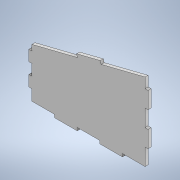
# Autodesk Inventor part: glass_separator
Saved by Autodesk Inventor 2020 (Build 240168000, 168)
## iProperties
Created: 2020-02-26
Part Number: glass_separator
Material: Generic
Document SubType Name: Modeling
Designer: udvarhelyi
Density: 1 g/cm^3
Appearance: Default
Author: udvarhelyi
Autodesk Inventor part; units mm, degrees
ref_plane "YZ Plane" through (0, 0, 0) normal (1, 0, 0) x (0, 1, 0)
ref_plane "XZ Plane" through (0, 0, 0) normal (0, 1, 0) x (-1, 0, 0)
ref_plane "XY Plane" through (0, 0, 0) normal (0, 0, 1) x (1, 0, 0)
sketch "Sketch1" plane through (0, 0, 0) normal (0, 0, 1) x (1, 0, 0)
  line L0 (14.8597, 70) -> (-9.1403, 64)
  line L1 (59.8597, 68) -> (62.8597, 68)
  line L2 (62.8597, 68) -> (62.8597, 51)
  line L3 (62.8597, 17) -> (59.8597, 17)
  line L4 (59.8597, 51) -> (62.8597, 51)
  line L5 (62.8597, 34) -> (62.8597, 17)
  line L6 (-54.1403, 22) -> (-57.1403, 22)
  line L7 (-57.1403, 22) -> (-57.1403, 11)
  line L8 (-57.1403, 11) -> (-54.1403, 11)
  line L9 (-54.1403, 44) -> (-57.1403, 44)
  line L10 (-57.1403, 44) -> (-57.1403, 33)
  line L11 (-57.1403, 33) -> (-54.1403, 33)
  line L12 (-8.5403, 0) -> (-8.5403, -3)
  line L13 (-8.5403, -3) -> (-31.3403, -3)
  line L14 (-31.3403, -3) -> (-31.3403, 0)
  line L15 (32.3597, 0) -> (37.0597, 0)
  line L16 (37.0597, 0) -> (37.0597, -3)
  line L17 (37.0597, -3) -> (14.2597, -3)
  line L18 (14.2597, -3) -> (14.2597, 0)
  line L19 (14.8597, 70) -> (15.5873, 67.0896)
  line L20 (-9.1403, 64) -> (-8.4127, 61.0896)
  line L21 (-54.1403, 22) -> (-54.1403, 33)
  line L22 (59.8597, 17) -> (59.8597, 0)
  line L23 (59.8597, 78.1577) -> (59.8597, 68)
  line L24 (59.8597, 34) -> (59.8597, 51)
  line L25 (-54.1403, 0) -> (-31.3403, 0)
  line L26 (-8.5403, 0) -> (14.2597, 0)
  line L27 (37.0597, 0) -> (59.8597, 0)
  line L28 (-54.1403, 49.6577) -> (-54.1403, 44)
  line L29 (-54.1403, 33) -> (-54.1403, 22)
  line L30 (-54.1403, 33) -> (-54.1403, 22)
  line L31 (-54.1403, 11) -> (-54.1403, 0)
  line L32 (14.8597, 70) -> (-57.1403, 52) construction
  line L33 (-57.1403, 44) -> (-57.1403, 60) construction
  line L34 (-54.1403, 49.6577) -> (-8.4127, 61.0896)
  line L35 (15.5873, 67.0896) -> (59.8597, 78.1577)
  line L36 (59.8597, 34) -> (62.8597, 34)
  line L37 (14.8597, 70) -> (98.136, 90.8191) construction
  line L38 (62.8597, 68) -> (62.8597, 104.4948) construction
  point P0 (0, 0)
  point P1 (62.8597, 82)
  dimension "d3" = 11
  dimension "d4" = 0
  dimension "d5" = 55
  dimension "d6" = 3
  dimension "d8" = 8.5403
  dimension "d9" = 22.8
  dimension "d10" = 3
  dimension "d11" = 3
  dimension "d12" = 114
  dimension "d13" = 24.7386
  dimension "d14" = 3
  dimension "d17" = 17
  dimension "d20" = 22.8
  dimension "d21" = 22.8
  dimension "d22" = 22.8
  dimension "d23" = 82
  dimension "d24" = 48
  dimension "d25" = 48
  dimension "d26" = 17
  dimension "d27" = 11
  constraints: 78 end point, 18 collinear, 10 horizontal, 8 perpendicular, 8 vertical, 7 point on line, 6 parallel, 2 midpoint
  measures "d3" distance of L6.end L7.end
  measures "d4" distance from line of L26 point (0, 0)
  measures "d5" distance from line of L13 point (-57.14, 52)
  measures "d6" distance of L13.end L14.end
  measures "d8" distance from line of L12 point (0, 0)
  measures "d9" distance of L12.end L13.end
  measures "d10" distance of L7.end L8.end
  measures "d11" distance of L3.start L3.end
  measures "d12" distance between parallel lines of L31 L22
  measures "d13" distance between parallel lines of L19 L20
  measures "d14" distance between parallel lines of L35 L0
  measures "d17" distance of L1.end L2.end
  measures "d20" distance of L25.start L14.end
  measures "d21" distance of L12.start L18.end
  measures "d22" distance of L15.end L22.end
  measures "d23" vertical distance of L22.end point (62.86, 82)
  measures "d24" horizontal distance of point (62.86, 82) L0.start
  measures "d25" horizontal distance of L0.end L32.end
  measures "d26" distance of L24.start L4.start
  measures "d27" distance of L6.start L11.end
extrude "Extrusion1" add sketch "Sketch1" along normal blind 3
equation "\"d6\" = tt"
equation "\"d9\" = -0.4 * tt + 0.2 * ht + 2 * tol"
equation "\"d10\" = tt"
equation "\"d11\" = tt"
equation "\"d12\" = -2 * tt + ht"
equation "\"d13\" = 0.2 * d"
equation "\"d14\" = tt"
equation "\"d24\" = d25"
equation "\"d18\" = tt"
equation "\"d0\" = tt"
equation "\"tt\" = 3"
equation "\"tol\" = 0"
equation "\"tiroir\" = 1"
equation "\"nHoles\" = 4"
equation "\"shelfH\" = 35"
equation "\"ht\" = 120"
equation "\"d\" = 123.693169"
body "Solid1"
